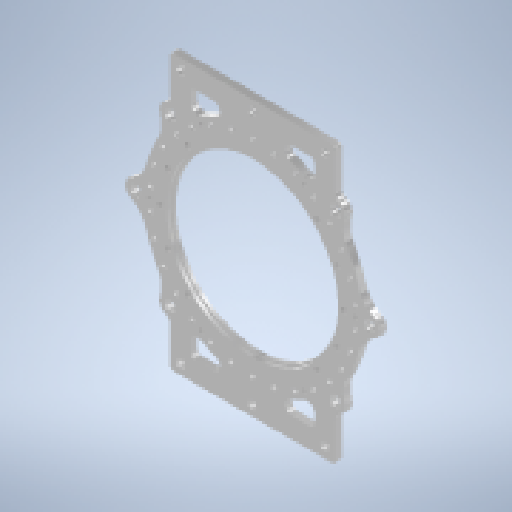
# Autodesk Inventor part: ベース板_出力側
Saved by Autodesk Inventor 2024 (Build 280153000, 153)
## iProperties
Created: 2023-05-29
Part Number: ベース板_出力側
Material: アルミニウム 6061
Document SubType Name: Modeling
Designer: yuta2
Density: 2.7 g/cm^3
Appearance: アルミニウム - フラット
Mass: 177.556 g
Surface Area: 373.92 cm^2
Volume: 65.7615 cm^3
Author: yuta2
Autodesk Inventor part; units mm, degrees
ref_plane "YZ Plane" through (0, 0, 0) normal (1, 0, 0) x (0, 1, 0)
ref_plane "XZ Plane" through (0, 0, 0) normal (0, 1, 0) x (-1, 0, 0)
ref_plane "XY Plane" through (0, 0, 0) normal (0, 0, 1) x (1, 0, 0)
sketch "スケッチ1" plane through (0, 0, 0) normal (0, 0, 1) x (1, 0, 0)
  circle A0 centre (0, 0) radius 80
  dimension "d0" = 160
  constraints: 1 centre point, 1 coincident
  measures "d0" diameter of A0
extrude "押し出し1" add sketch "スケッチ1" along normal blind 5
sketch "スケッチ2" plane through (0, 0, 5) normal (0, 0, 1) x (1, 0, 0)
  circle A0 centre (0, 0) radius 60.5
  dimension "d3" = 121
  constraints: 1 centre point, 1 coincident
  measures "d3" diameter of A0
extrude "押し出し2" cut sketch "スケッチ2" against normal through all
sketch "スケッチ3" plane through (0, 0, 5) normal (0, 0, 1) x (1, 0, 0)
  point P0 (0, 0)
  point P1 (0, 75)
  dimension "d6" = 75
  constraints: 1 vertical alignment
  measures "d6" distance of point (0, 0) point (0, 75)
hole "穴1" at (0, 75, 5) direction (0, 0, -1) diameter 4 end through all
pattern_circular "円形状パターン1" count 30 over 360 about axis through (0, 0, 0) along (0, 0, 1) of "穴1"
sketch "スケッチ4" plane through (0, 0, 5) normal (0, 0, 1) x (1, 0, 0)
  circle A0 centre (0, 0) radius 62.5
  dimension "d17" = 125
  constraints: 1 centre point, 1 coincident
  measures "d17" diameter of A0
extrude "押し出し3" cut sketch "スケッチ4" against normal blind 2.5
sketch "スケッチ5" plane through (0, 0, 5) normal (0, 0, 1) x (1, 0, 0)
  circle A0 centre (66.5, 0) radius 4
  circle A1 centre (61.438, 25.4484) radius 4
  circle A2 centre (47.0226, 47.0226) radius 4
  circle A3 centre (25.4484, 61.438) radius 4
  circle A4 centre (0, 66.5) radius 4
  circle A5 centre (-25.4484, 61.438) radius 4
  circle A6 centre (-47.0226, 47.0226) radius 4
  circle A7 centre (-61.438, 25.4484) radius 4
  circle A8 centre (-66.5, 0) radius 4
  circle A9 centre (-61.438, -25.4484) radius 4
  circle A10 centre (-47.0226, -47.0226) radius 4
  circle A11 centre (-25.4484, -61.438) radius 4
  circle A12 centre (0, -66.5) radius 4
  circle A13 centre (25.4484, -61.438) radius 4
  circle A14 centre (47.0226, -47.0226) radius 4
  circle A15 centre (61.438, -25.4484) radius 4
  point P0 (0, 0)
  dimension "d20" = 8
  dimension "d21" = 66.5
  dimension "d24" = 360
  constraints: 16 centre point, 10 coincident, 1 horizontal alignment, 33 other
  measures "d20" diameter of A0
  measures "d21" distance of point (0, 0) A0.centre
hole "穴2" at (47.0226, 47.0226, 5) at (61.438, 25.4484, 5) at (66.5, 0, 5) at (61.438, -25.4484, 5) at (47.0226, -47.0226, 5) at (-47.0226, -47.0226, 5) at (-61.438, -25.4484, 5) at (-66.5, 0, 5) at (-61.438, 25.4484, 5) at (-47.0226, 47.0226, 5) direction (0, 0, -1) diameter 4 end through all
thread "ねじ1" size "M4x0.7" class "6H" standard "ANSI Metric M Profile" full length
thread "ねじ2" size "M4x0.7" class "6H" standard "ANSI Metric M Profile" full length
thread "ねじ3" size "M4x0.7" class "6H" standard "ANSI Metric M Profile" full length
thread "ねじ4" size "M4x0.7" class "6H" standard "ANSI Metric M Profile" full length
thread "ねじ5" size "M4x0.7" class "6H" standard "ANSI Metric M Profile" full length
thread "ねじ6" size "M4x0.7" class "6H" standard "ANSI Metric M Profile" full length
thread "ねじ7" size "M4x0.7" class "6H" standard "ANSI Metric M Profile" full length
thread "ねじ8" size "M4x0.7" class "6H" standard "ANSI Metric M Profile" full length
thread "ねじ9" size "M4x0.7" class "6H" standard "ANSI Metric M Profile" full length
thread "ねじ10" size "M4x0.7" class "6H" standard "ANSI Metric M Profile" full length
sketch "スケッチ6" plane through (0, 0, 5) normal (0, 0, 1) x (1, 0, 0)
  point P0 (0, 0)
  point P1 (75, 0)
  dimension "d53" = 75
  constraints: 1 horizontal alignment
  measures "d53" distance of point (0, 0) point (75, 0)
hole "穴3" at (75, 0, 5) direction (0, 0, -1) diameter 3 end through all
thread "ねじ11" size "M3x0.5" class "6H" standard "ANSI Metric M Profile" full length
pattern_circular "円形状パターン2" count 6 over 360 about axis through (0, 0, 0) along (0, 0, 1) of "穴3"
sketch "スケッチ7" plane through (0, 0, 5) normal (0, 0, 1) x (1, 0, 0)
  circle A0 centre (-85, 0) radius 7.5
  circle A1 centre (0, 0) radius 80 projected
  arc A2 (-77.5, -19.8431) -> (-88.2386, -6.7647) centre (-96.875, -24.8039) ccw
  circle A3 centre (0, 0) radius 80 projected
  line L0 (0, 0) -> (-50.2153, 0)
  arc A4 (-88.2386, 6.7647) -> (-77.5, 19.8431) centre (-96.875, 24.8039) ccw
  arc A5 (-40.7696, -68.832) -> (-57.6108, -67.1775) centre (-50.962, -86.04) ccw
  circle A6 centre (-60.1041, -60.1041) radius 7.5
  arc A7 (-67.1775, -57.6108) -> (-68.832, -40.7696) centre (-86.04, -50.962) ccw
  arc A8 (-57.6108, 67.1775) -> (-40.7696, 68.832) centre (-50.962, 86.04) ccw
  circle A9 centre (-60.1041, 60.1041) radius 7.5
  arc A10 (-68.832, 40.7696) -> (-67.1775, 57.6108) centre (-86.04, 50.962) ccw
  point P0 (-40.7696, 68.832)
  point P1 (-67.1775, 57.6108)
  point P2 (-88.2386, 6.7647)
  point P3 (-40.7696, -68.832)
  point P4 (-67.1775, -57.6108)
  dimension "d66" = 15
  dimension "d67" = 85
  dimension "d68" = 20
  dimension "d71" = 45
  constraints: 12 point on circle, 10 symmetric about line, 6 centre point, 2 end point, 2 horizontal, 1 horizontal alignment, 28 other
  measures "d67" distance of point (-85, 0) point (0, 0)
  measures "d68" radius of A2
extrude "押し出し4" add sketch "スケッチ7" against normal blind 5 contours A0 A1 | A4 A1 A0 | A0 A1 A2 | A10 A9 A1 | A1 A6 A7 | A9 A1 | A1 A6 | A9 A8 A1 | A1 A5 A6 picked at (-84.1336, -0.3115) picked at (-59.7117, 59.2712) picked at (-59.7117, -59.2712)
sketch "スケッチ8" plane through (0, 0, 5) normal (0, 0, 1) x (1, 0, 0)
  arc A0 (-67.1775, -57.6108) -> (-57.6108, -67.1775) centre (-60.1041, -60.1041) ccw projected
  arc A1 (-88.2386, 6.7647) -> (-88.2386, -6.7647) centre (-85, 0) ccw projected
  arc A2 (-57.6108, 67.1775) -> (-67.1775, 57.6108) centre (-60.1041, 60.1041) ccw projected
  point P0 (0, 0)
  constraints: 3 coincident
hole "穴4" at (-60.1041, -60.1041, 5) at (-85, 0, 5) at (-60.1041, 60.1041, 5) direction (0, 0, -1) diameter 8 end through all
pattern_circular "円形状パターン3" count 2 over 360 about axis through (0, 0, 0) along (0, 0, 1) of "押し出し4", "穴4"
sketch "スケッチ9" plane through (0, 0, 5) normal (0, 0, 1) x (1, 0, 0)
  line L0 (-60, -100) -> (60, -100)
  line L1 (60, -100) -> (60, 100)
  line L2 (60, 100) -> (-60, 100)
  line L3 (-60, 100) -> (-60, -100)
  circle A0 centre (60.1041, -60.1041) radius 4 projected
  circle A1 centre (60.1041, 60.1041) radius 4 projected
  circle A2 centre (85, 0) radius 4 projected
  circle A3 centre (-60.1041, 60.1041) radius 4 projected
  circle A4 centre (-85, 0) radius 4 projected
  circle A5 centre (-60.1041, -60.1041) radius 4 projected
  circle A6 centre (37.5, -64.9519) radius 1.5 projected
  circle A7 centre (-37.5, -64.9519) radius 1.5 projected
  circle A8 centre (-75, 0) radius 1.5 projected
  circle A9 centre (-37.5, 64.9519) radius 1.5 projected
  circle A10 centre (37.5, 64.9519) radius 1.5 projected
  circle A11 centre (75, 0) radius 1.5 projected
  circle A12 centre (-47.0226, 47.0226) radius 2 projected
  circle A13 centre (-61.438, 25.4484) radius 2 projected
  circle A14 centre (-66.5, 0) radius 2 projected
  circle A15 centre (-61.438, -25.4484) radius 2 projected
  circle A16 centre (-47.0226, -47.0226) radius 2 projected
  circle A17 centre (47.0226, -47.0226) radius 2 projected
  circle A18 centre (61.438, -25.4484) radius 2 projected
  circle A19 centre (66.5, 0) radius 2 projected
  circle A20 centre (61.438, 25.4484) radius 2 projected
  circle A21 centre (47.0226, 47.0226) radius 2 projected
  circle A22 centre (0, 0) radius 62.5 projected
  circle A23 centre (15.5934, 73.3611) radius 2 projected
  circle A24 centre (30.5052, 68.5159) radius 2 projected
  circle A25 centre (44.0839, 60.6763) radius 2 projected
  circle A26 centre (55.7359, 50.1848) radius 2 projected
  circle A27 centre (64.9519, 37.5) radius 2 projected
  circle A28 centre (71.3292, 23.1763) radius 2 projected
  circle A29 centre (74.5891, 7.8396) radius 2 projected
  circle A30 centre (74.5891, -7.8396) radius 2 projected
  circle A31 centre (71.3292, -23.1763) radius 2 projected
  circle A32 centre (64.9519, -37.5) radius 2 projected
  circle A33 centre (55.7359, -50.1848) radius 2 projected
  circle A34 centre (44.0839, -60.6763) radius 2 projected
  circle A35 centre (30.5052, -68.5159) radius 2 projected
  circle A36 centre (15.5934, -73.3611) radius 2 projected
  circle A37 centre (0, -75) radius 2 projected
  circle A38 centre (-15.5934, -73.3611) radius 2 projected
  circle A39 centre (-30.5052, -68.5159) radius 2 projected
  circle A40 centre (-44.0839, -60.6763) radius 2 projected
  circle A41 centre (-55.7359, -50.1848) radius 2 projected
  circle A42 centre (-64.9519, -37.5) radius 2 projected
  circle A43 centre (-71.3292, -23.1763) radius 2 projected
  circle A44 centre (-74.5891, -7.8396) radius 2 projected
  circle A45 centre (-74.5891, 7.8396) radius 2 projected
  circle A46 centre (-71.3292, 23.1763) radius 2 projected
  circle A47 centre (-64.9519, 37.5) radius 2 projected
  circle A48 centre (-55.7359, 50.1848) radius 2 projected
  circle A49 centre (-44.0839, 60.6763) radius 2 projected
  circle A50 centre (-30.5052, 68.5159) radius 2 projected
  circle A51 centre (-15.5934, 73.3611) radius 2 projected
  circle A52 centre (0, 75) radius 2 projected
  arc A53 (-40.7696, -68.832) -> (40.7696, -68.832) centre (0, 0) ccw projected
  arc A54 (57.6108, -67.1775) -> (40.7696, -68.832) centre (50.962, -86.04) ccw projected
  arc A55 (57.6108, -67.1775) -> (67.1775, -57.6108) centre (60.1041, -60.1041) ccw projected
  arc A56 (68.832, -40.7696) -> (67.1775, -57.6108) centre (86.04, -50.962) ccw projected
  arc A57 (68.832, -40.7696) -> (77.5, -19.8431) centre (0, 0) ccw projected
  arc A58 (88.2386, -6.7647) -> (77.5, -19.8431) centre (96.875, -24.8039) ccw projected
  arc A59 (88.2386, -6.7647) -> (88.2386, 6.7647) centre (85, 0) ccw projected
  arc A60 (77.5, 19.8431) -> (88.2386, 6.7647) centre (96.875, 24.8039) ccw projected
  arc A61 (77.5, 19.8431) -> (68.832, 40.7696) centre (0, 0) ccw projected
  arc A62 (67.1775, 57.6108) -> (68.832, 40.7696) centre (86.04, 50.962) ccw projected
  arc A63 (67.1775, 57.6108) -> (57.6108, 67.1775) centre (60.1041, 60.1041) ccw projected
  arc A64 (40.7696, 68.832) -> (57.6108, 67.1775) centre (50.962, 86.04) ccw projected
  arc A65 (40.7696, 68.832) -> (-40.7696, 68.832) centre (0, 0) ccw projected
  arc A66 (-57.6108, 67.1775) -> (-40.7696, 68.832) centre (-50.962, 86.04) ccw projected
  arc A67 (-57.6108, 67.1775) -> (-67.1775, 57.6108) centre (-60.1041, 60.1041) ccw projected
  arc A68 (-68.832, 40.7696) -> (-67.1775, 57.6108) centre (-86.04, 50.962) ccw projected
  arc A69 (-68.832, 40.7696) -> (-77.5, 19.8431) centre (0, 0) ccw projected
  arc A70 (-88.2386, 6.7647) -> (-77.5, 19.8431) centre (-96.875, 24.8039) ccw projected
  arc A71 (-88.2386, 6.7647) -> (-88.2386, -6.7647) centre (-85, 0) ccw projected
  arc A72 (-77.5, -19.8431) -> (-88.2386, -6.7647) centre (-96.875, -24.8039) ccw projected
  arc A73 (-77.5, -19.8431) -> (-68.832, -40.7696) centre (0, 0) ccw projected
  arc A74 (-67.1775, -57.6108) -> (-68.832, -40.7696) centre (-86.04, -50.962) ccw projected
  arc A75 (-67.1775, -57.6108) -> (-57.6108, -67.1775) centre (-60.1041, -60.1041) ccw projected
  arc A76 (-40.7696, -68.832) -> (-57.6108, -67.1775) centre (-50.962, -86.04) ccw projected
  line L4 (0, 0) -> (-66.5, 0)
  line L5 (0, 0) -> (0, 75)
  point P0 (-60, 67.6034)
  point P1 (60, 67.6034)
  point P2 (60, -67.6034)
  point P3 (-60, -67.6034)
  dimension "d85" = 200
  dimension "d86" = 120
  constraints: 12 end point, 2 horizontal, 2 parallel, 1 perpendicular, 1 vertical, 2 other
  measures "d85" distance of L2.end L0.start
  measures "d86" distance of L1.end L2.end
extrude "押し出し5" add sketch "スケッチ9" against normal blind 5 contours L3 A75 A76 A53 A54 A55 L1 L0 | L3 L2 L1 A63 A64 A65 A66 A67
sketch "スケッチ10" plane through (0, 0, 5) normal (0, 0, 1) x (1, 0, 0)
  line L0 (60, -100) -> (-60, -100) projected
  line L1 (0, -100) -> (0, 100) construction
  line L2 (-60, 100) -> (60, 100) projected
  line L3 (-60, -100) -> (-60, -67.6034) projected
  line L4 (-60, -92.5) -> (60, -92.5) construction
  line L5 (60, -67.6034) -> (60, -100) projected
  line L6 (0, 0) -> (-65.4143, 0)
  line L7 (0, -100) -> (0, 100)
  line L8 (-60, -67.6034) -> (-60, -100) projected
  line L9 (-60, -100) -> (60, -100) projected
  line L10 (0, 100) -> (0, -100) construction
  line L11 (-60, 92.5) -> (60, 92.5) construction
  point P0 (-52.5, -92.5)
  point P1 (52.5, -92.5)
  point P2 (0, -92.5)
  point P3 (-52.5, 92.5)
  point P4 (52.5, 92.5)
  point P5 (0, 92.5)
  dimension "d89" = 7.5
  dimension "d90" = 7.5
  constraints: 12 end point, 8 symmetric about line, 7 point on line, 4 midpoint, 1 horizontal, 1 perpendicular, 1 vertical
  measures "d89" distance from line of L8 point (-52.5, -92.5)
  measures "d90" distance between parallel lines of L9 L4
hole "穴5" at (-52.5, -92.5, 5) at (52.5, -92.5, 5) at (0, -92.5, 5) at (0, 92.5, 5) at (-52.5, 92.5, 5) at (52.5, 92.5, 5) direction (0, 0, -1) diameter 6 end through all
fillet "フィレット1" radius 5 4 edges at (-60, 67.6034, 2.5) (60, 67.6034, 2.5) (60, -67.6034, 2.5) (-60, -67.6034, 2.5)
fillet "フィレット2" radius 2 4 edges at (-60, 100, 2.5) (60, 100, 2.5) (60, -100, 2.5) (-60, -100, 2.5)
sketch "スケッチ11" plane through (0, 0, 5) normal (0, 0, 1) x (1, 0, 0)
  circle A0 centre (0, 0) radius 80
  arc A1 (-60, -98) -> (-58, -100) centre (-58, -98) ccw projected
  line L0 (-58, -100) -> (58, -100) projected
  arc A2 (58, -100) -> (60, -98) centre (58, -98) ccw projected
  line L1 (60, -98) -> (60, -71.6054) projected
  arc A3 (63.0416, -67.0049) -> (60, -71.6054) centre (65, -71.6054) ccw projected
  arc A4 (63.0416, -67.0049) -> (67.1775, -57.6108) centre (60.1041, -60.1041) ccw projected
  arc A5 (68.832, -40.7696) -> (67.1775, -57.6108) centre (86.04, -50.962) ccw projected
  arc A6 (68.832, -40.7696) -> (77.5, -19.8431) centre (0, 0) ccw projected
  arc A7 (88.2386, -6.7647) -> (77.5, -19.8431) centre (96.875, -24.8039) ccw projected
  arc A8 (88.2386, -6.7647) -> (88.2386, 6.7647) centre (85, 0) ccw projected
  arc A9 (77.5, 19.8431) -> (88.2386, 6.7647) centre (96.875, 24.8039) ccw projected
  arc A10 (77.5, 19.8431) -> (68.832, 40.7696) centre (0, 0) ccw projected
  arc A11 (67.1775, 57.6108) -> (68.832, 40.7696) centre (86.04, 50.962) ccw projected
  arc A12 (67.1775, 57.6108) -> (63.0416, 67.0049) centre (60.1041, 60.1041) ccw projected
  arc A13 (60, 71.6054) -> (63.0416, 67.0049) centre (65, 71.6054) ccw projected
  line L2 (60, 71.6054) -> (60, 98) projected
  arc A14 (60, 98) -> (58, 100) centre (58, 98) ccw projected
  line L3 (58, 100) -> (-58, 100) projected
  arc A15 (-58, 100) -> (-60, 98) centre (-58, 98) ccw projected
  line L4 (-60, 98) -> (-60, 71.6054) projected
  arc A16 (-63.0416, 67.0049) -> (-60, 71.6054) centre (-65, 71.6054) ccw projected
  arc A17 (-63.0416, 67.0049) -> (-67.1775, 57.6108) centre (-60.1041, 60.1041) ccw projected
  arc A18 (-68.832, 40.7696) -> (-67.1775, 57.6108) centre (-86.04, 50.962) ccw projected
  arc A19 (-68.832, 40.7696) -> (-77.5, 19.8431) centre (0, 0) ccw projected
  arc A20 (-88.2386, 6.7647) -> (-77.5, 19.8431) centre (-96.875, 24.8039) ccw projected
  arc A21 (-88.2386, 6.7647) -> (-88.2386, -6.7647) centre (-85, 0) ccw projected
  arc A22 (-77.5, -19.8431) -> (-88.2386, -6.7647) centre (-96.875, -24.8039) ccw projected
  arc A23 (-77.5, -19.8431) -> (-68.832, -40.7696) centre (0, 0) ccw projected
  arc A24 (-67.1775, -57.6108) -> (-68.832, -40.7696) centre (-86.04, -50.962) ccw projected
  arc A25 (-67.1775, -57.6108) -> (-63.0416, -67.0049) centre (-60.1041, -60.1041) ccw projected
  arc A26 (-60, -71.6054) -> (-63.0416, -67.0049) centre (-65, -71.6054) ccw projected
  line L5 (-60, -71.6054) -> (-60, -98) projected
  circle A27 centre (52.5, 92.5) radius 3 projected
  circle A28 centre (-52.5, 92.5) radius 3 projected
  circle A29 centre (0, 92.5) radius 3 projected
  circle A30 centre (0, -92.5) radius 3 projected
  circle A31 centre (52.5, -92.5) radius 3 projected
  circle A32 centre (-52.5, -92.5) radius 3 projected
  circle A33 centre (60.1041, -60.1041) radius 4 projected
  circle A34 centre (60.1041, 60.1041) radius 4 projected
  circle A35 centre (85, 0) radius 4 projected
  circle A36 centre (-60.1041, 60.1041) radius 4 projected
  circle A37 centre (-85, 0) radius 4 projected
  circle A38 centre (-60.1041, -60.1041) radius 4 projected
  circle A39 centre (37.5, -64.9519) radius 1.5 projected
  circle A40 centre (-37.5, -64.9519) radius 1.5 projected
  circle A41 centre (-75, 0) radius 1.5 projected
  circle A42 centre (-37.5, 64.9519) radius 1.5 projected
  circle A43 centre (37.5, 64.9519) radius 1.5 projected
  circle A44 centre (75, 0) radius 1.5 projected
  circle A45 centre (-47.0226, 47.0226) radius 2 projected
  circle A46 centre (-61.438, 25.4484) radius 2 projected
  circle A47 centre (-66.5, 0) radius 2 projected
  circle A48 centre (-61.438, -25.4484) radius 2 projected
  circle A49 centre (-47.0226, -47.0226) radius 2 projected
  circle A50 centre (47.0226, -47.0226) radius 2 projected
  circle A51 centre (61.438, -25.4484) radius 2 projected
  circle A52 centre (66.5, 0) radius 2 projected
  circle A53 centre (61.438, 25.4484) radius 2 projected
  circle A54 centre (47.0226, 47.0226) radius 2 projected
  circle A55 centre (0, 0) radius 62.5 projected
  circle A56 centre (15.5934, 73.3611) radius 2 projected
  circle A57 centre (30.5052, 68.5159) radius 2 projected
  circle A58 centre (44.0839, 60.6763) radius 2 projected
  circle A59 centre (55.7359, 50.1848) radius 2 projected
  circle A60 centre (64.9519, 37.5) radius 2 projected
  circle A61 centre (71.3292, 23.1763) radius 2 projected
  circle A62 centre (74.5891, 7.8396) radius 2 projected
  circle A63 centre (74.5891, -7.8396) radius 2 projected
  circle A64 centre (71.3292, -23.1763) radius 2 projected
  circle A65 centre (64.9519, -37.5) radius 2 projected
  circle A66 centre (55.7359, -50.1848) radius 2 projected
  circle A67 centre (44.0839, -60.6763) radius 2 projected
  circle A68 centre (30.5052, -68.5159) radius 2 projected
  circle A69 centre (15.5934, -73.3611) radius 2 projected
  circle A70 centre (0, -75) radius 2 projected
  circle A71 centre (-15.5934, -73.3611) radius 2 projected
  circle A72 centre (-30.5052, -68.5159) radius 2 projected
  circle A73 centre (-44.0839, -60.6763) radius 2 projected
  circle A74 centre (-55.7359, -50.1848) radius 2 projected
  circle A75 centre (-64.9519, -37.5) radius 2 projected
  circle A76 centre (-71.3292, -23.1763) radius 2 projected
  circle A77 centre (-74.5891, -7.8396) radius 2 projected
  circle A78 centre (-74.5891, 7.8396) radius 2 projected
  circle A79 centre (-71.3292, 23.1763) radius 2 projected
  circle A80 centre (-64.9519, 37.5) radius 2 projected
  circle A81 centre (-55.7359, 50.1848) radius 2 projected
  circle A82 centre (-44.0839, 60.6763) radius 2 projected
  circle A83 centre (-30.5052, 68.5159) radius 2 projected
  circle A84 centre (-15.5934, 73.3611) radius 2 projected
  circle A85 centre (0, 75) radius 2 projected
  line L6 (-60, 100) -> (60, 100)
  line L7 (60, 100) -> (60, -100)
  line L8 (60, -100) -> (-60, -100)
  line L9 (-60, -100) -> (-60, 100)
  line L10 (-58, -100) -> (58, -100) projected
  line L11 (58, 100) -> (-58, 100) projected
  line L12 (-60, 98) -> (-60, 71.6054) projected
  line L13 (60, 71.6054) -> (60, 98) projected
  line L14 (-42, 85) -> (45, 85)
  line L15 (45, 85) -> (45, -85)
  line L16 (45, -85) -> (-45, -85)
  line L17 (-45, -85) -> (-45, 82)
  arc A86 (-45, 75) -> (-37.6471, 70.5882) centre (-40, 75) ccw
  arc A87 (-27.0332, 75.2941) -> (-28.7228, 85) centre (-28.7228, 80) ccw
  arc A88 (-42, 85) -> (-45, 82) centre (-42, 82) ccw
  line L18 (0, -75) -> (0, 75)
  line L19 (0, 75) -> (-60, 0)
  line L20 (0, 0) -> (-60, 0)
  arc A89 (37.6471, 70.5882) -> (45, 75) centre (40, 75) ccw
  arc A90 (28.7228, 85) -> (27.0332, 75.2941) centre (28.7228, 80) ccw
  arc A91 (45, 82) -> (42, 85) centre (42, 82) ccw
  arc A92 (-37.6471, -70.5882) -> (-45, -75) centre (-40, -75) ccw
  arc A93 (-28.7228, -85) -> (-27.0332, -75.2941) centre (-28.7228, -80) ccw
  arc A94 (-45, -82) -> (-42, -85) centre (-42, -82) ccw
  arc A95 (45, -75) -> (37.6471, -70.5882) centre (40, -75) ccw
  arc A96 (27.0332, -75.2941) -> (28.7228, -85) centre (28.7228, -80) ccw
  arc A97 (42, -85) -> (45, -82) centre (42, -82) ccw
  point P0 (28.7228, 85)
  point P1 (27.0332, 75.2941)
  point P2 (45, 75)
  point P3 (45, -75)
  point P4 (37.6471, -70.5882)
  point P5 (28.7228, -85)
  point P6 (42, -85)
  point P7 (-27.0332, -75.2941)
  point P8 (-45, -75)
  point P9 (-42, -85)
  dimension "d100" = 160
  dimension "d101" = 15
  dimension "d102" = 5
  dimension "d103" = 5
  dimension "d104" = 3
  constraints: 27 symmetric about line, 26 point on circle, 22 end point, 13 centre point, 6 tangent, 4 collinear, 4 parallel, 3 perpendicular, 2 point on line, 1 coincident, 1 horizontal, 1 midpoint, 1 vertical, 12 other
  measures "d100" diameter of A0
  measures "d101" distance between parallel lines of L9 L17
  measures "d102" radius of A86
  measures "d103" radius of A87
  measures "d104" radius of A88
extrude "押し出し6" cut sketch "スケッチ11" against normal blind 5 contours A0 A90 L14 A91 L15 A89 | A95 L15 A97 L16 A96 A0 | A0 A86 L17 A88 L14 A87 | A93 L16 A94 L17 A92 A0
equation "\"d6\" = 0.5 * D"
equation "\"d53\" = 0.5 * D"
equation "\"D\" = 150"
